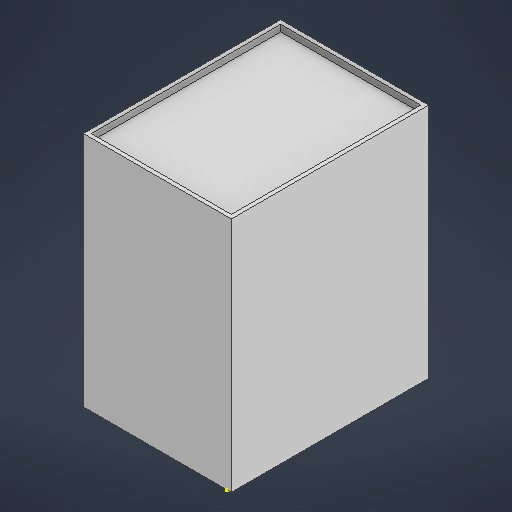
# Autodesk Inventor part: box
Saved by Autodesk Inventor 2027.1 (Build 311270010, 270A)
## iProperties
Created: 2026-10-02
Part Number: box
Material: Generic
Document SubType Name: Modeling
Designer: Arik
Density: 1 g/cm^3
Appearance: Default
Author: Arik
Autodesk Inventor part; units mm, degrees
ref_plane "YZ Plane" through (0, 0, 0) normal (1, 0, 0) x (0, 1, 0)
ref_plane "XZ Plane" through (0, 0, 0) normal (0, 1, 0) x (-1, 0, 0)
ref_plane "XY Plane" through (0, 0, 0) normal (0, 0, 1) x (1, 0, 0)
sketch "Sketch1" plane through (0, 0, 0) normal (0, 1, 0) x (-1, 0, 0)
  line L0 (0, 0) -> (450, 0)
  line L1 (450, 0) -> (450, -600)
  line L2 (450, -600) -> (0, -600)
  line L3 (0, -600) -> (0, 0)
  dimension "d0" = 450
  dimension "d1" = 600
  constraints: 8 end point, 2 parallel, 1 horizontal, 1 perpendicular
  measures "d0" distance of L1.end L2.end
  measures "d1" distance of L0.end L1.end
extrude "Extrusion1" add sketch "Sketch1" along normal blind 12
sketch "Sketch2" plane through (0, 12, 0) normal (0, 1, 0) x (1, 0, 0)
  line L0 (0, 0) -> (0, 600) projected
  line L1 (-450, 600) -> (-450, 0) projected
  line L2 (0, 600) -> (-450, 600)
  line L3 (-450, 600) -> (-450, 0)
  line L4 (-450, 0) -> (0, 0)
  line L5 (0, 0) -> (0, 600)
  line L6 (-438, 588) -> (-12, 588)
  line L7 (-12, 588) -> (-12, 12)
  line L8 (-12, 12) -> (-438, 12)
  line L9 (-438, 12) -> (-438, 588)
  dimension "d4" = 12
  constraints: 16 end point, 4 parallel, 2 perpendicular, 1 horizontal, 3 other
  measures "d4" distance between parallel lines of L2 L6
extrude "Extrusion2" add sketch "Sketch2" along normal blind 708
sketch "Sketch3" plane through (-450, 0, -600) normal (-1, 0, 0) x (0, 0, 1)
  line L0 (0, 0) -> (40, 0)
  line L1 (40, 0) -> (40, 100)
  line L2 (40, 100) -> (0, 100)
  line L3 (0, 100) -> (0, 0)
  line L4 (600, 0) -> (560, 0)
  line L5 (560, 0) -> (560, 100)
  line L6 (560, 100) -> (600, 100)
  line L7 (600, 100) -> (600, 0)
  line L8 (600, 720) -> (560, 720)
  line L9 (560, 720) -> (560, 620)
  line L10 (560, 620) -> (600, 620)
  line L11 (600, 620) -> (600, 720)
  line L12 (40, 100) -> (560, 100)
  line L13 (560, 100) -> (560, 620)
  line L14 (560, 620) -> (40, 620)
  line L15 (40, 620) -> (40, 100)
  dimension "d7" = 40
  dimension "d8" = 100
  dimension "d9" = 40
  dimension "d10" = 100
  dimension "d11" = 40
  dimension "d12" = 100
  constraints: 32 end point, 8 parallel, 4 horizontal, 4 perpendicular, 1 point on line
  measures "d7" distance of L2.end L1.end
  measures "d8" distance of L1.end L0.end
  measures "d9" distance of L5.end L6.end
  measures "d10" distance of L4.end L5.end
  measures "d11" distance of L10.end L9.end
  measures "d12" distance of L9.end L8.end
extrude "Extrusion3" cut sketch "Sketch3" against normal blind 12 contours L15 L14 L13 L12
sketch "Sketch4" plane through (-12, 12, -588) normal (-1, 0, 0) x (0, 0, 1)
  point P0 (588, -12)
sketch "Sketch5" plane through (-12, 12, -588) normal (-1, 0, 0) x (0, 0, 1)
  line L0 (0, 0) -> (0, 708) projected
  line L1 (0, 708) -> (0, 688)
  line L2 (576, 0) -> (576, 708) projected
  line L3 (0, 688) -> (576, 688)
  line L4 (576, 688) -> (576, 676)
  line L5 (576, 676) -> (0, 676)
  line L6 (0, 676) -> (0, 688)
  point P0 (588, -12)
  dimension "d15" = 20
  dimension "d16" = 12
  constraints: 10 end point, 2 parallel, 2 point on line, 1 horizontal, 1 perpendicular
  measures "d15" distance of L0.end L1.end
  measures "d16" distance of L3.end L4.end
extrude "Extrusion4" add sketch "Sketch5" along normal up to surface (438 mm away)
body "Solid1"
